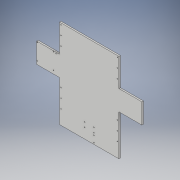
# Autodesk Inventor part: 20Gen2PlatePart
Saved by Autodesk Inventor 2019 (Build 230136000, 136)
## iProperties
Created: 2017-12-06
Part Number: 20Gen2PlatePart
Material: Generic
Document SubType Name: Modeling
Designer: User
Density: 1 g/cm^3
Appearance: Default
Mass: 688.034 g
Surface Area: 2294.14 cm^2
Volume: 688.034 cm^3
Author: User
Autodesk Inventor part; units mm, degrees
ref_plane "YZ Plane" through (0, 0, 0) normal (1, 0, 0) x (0, 1, 0)
ref_plane "XZ Plane" through (0, 0, 0) normal (0, 1, 0) x (-1, 0, 0)
ref_plane "XY Plane" through (0, 0, 0) normal (0, 0, 1) x (1, 0, 0)
ref_plane "Work Plane32" through (254, 330.2, 0) normal (0, 0, -1) x (-1, 0, 0)
sketch "Sketch36" plane through (254, 330.2, 0) normal (0, 0, -1) x (-1, 0, 0)
  line L0 (254, -363.855) -> (254, -196.85) projected
  line L1 (0, 0) -> (0, -114.3) projected
  line L2 (254, -363.855) -> (0, -363.855)
  line L3 (0, -363.855) -> (0, 0)
  line L4 (0, 0) -> (254, 0)
  line L5 (254, 0) -> (254, -363.855)
  line L6 (342.9, -196.85) -> (342.9, -114.3) projected
  line L7 (342.9, -196.85) -> (254, -196.85)
  line L8 (254, -196.85) -> (254, -114.3)
  line L9 (254, -114.3) -> (342.9, -114.3)
  line L10 (342.9, -114.3) -> (342.9, -196.85)
  line L11 (-31.75, -363.855) -> (254, -363.855) projected
  line L12 (0, -314.325) -> (0, -196.85) projected
  line L13 (-31.75, -363.855) -> (0, -363.855)
  line L14 (0, -363.855) -> (0, -314.325)
  line L15 (0, -314.325) -> (-31.75, -314.325)
  line L16 (-31.75, -314.325) -> (-31.75, -363.855)
  line L17 (0, -196.85) -> (-88.9, -196.85)
  line L18 (-88.9, -196.85) -> (-88.9, -114.3)
  line L19 (-88.9, -114.3) -> (0, -114.3)
  line L20 (0, -114.3) -> (0, -196.85)
  dimension "d412" = 82.55
  dimension "d413" = 254
  dimension "d414" = 31.75
  constraints: 32 end point, 8 parallel, 4 horizontal, 4 perpendicular, 1 point on line
  measures "d412" distance between parallel lines of L9 L7
  measures "d413" distance between parallel lines of L5 L1
  measures "d414" distance between parallel lines of L3 L16
extrude "Extrusion20" add sketch "Sketch36" along normal blind 6.35
ref_plane "Work Plane28" through (254, 330.2, -6.35) normal (0, 0, -1) x (-1, 0, 0)
sketch "Sketch38" plane through (254, 330.2, -6.35) normal (0, 0, -1) x (-1, 0, 0)
  circle A0 centre (273.685, -183.515) radius 1.778 projected
  circle A1 centre (273.685, -183.515) radius 1.778
  circle A2 centre (339.725, -183.515) radius 1.778 projected
  circle A3 centre (339.725, -183.515) radius 1.778
  circle A4 centre (339.725, -117.475) radius 1.778 projected
  circle A5 centre (339.725, -117.475) radius 1.778
  circle A6 centre (273.685, -117.475) radius 1.778 projected
  circle A7 centre (273.685, -117.475) radius 1.778
  circle A8 centre (263.1059, -119.0625) radius 1.778 projected
  circle A9 centre (263.1059, -119.0625) radius 1.778
  circle A10 centre (107.95, -332.105) radius 1.905 projected
  circle A11 centre (107.95, -332.105) radius 1.905
  circle A12 centre (107.95, -322.58) radius 1.905 projected
  circle A13 centre (107.95, -322.58) radius 1.905
  circle A14 centre (107.95, -303.53) radius 1.905 projected
  circle A15 centre (107.95, -303.53) radius 1.905
  circle A16 centre (107.95, -357.505) radius 1.905 projected
  circle A17 centre (107.95, -357.505) radius 1.905
  circle A18 centre (146.05, -303.53) radius 1.905 projected
  circle A19 centre (146.05, -303.53) radius 1.905
  circle A20 centre (146.05, -322.58) radius 1.905 projected
  circle A21 centre (146.05, -322.58) radius 1.905
  constraints: 11 centre point, 11 coincident
extrude "Extrusion21" cut sketch "Sketch38" against normal blind 6.35
sketch "Sketch39" plane through (254, 330.2, -6.35) normal (0, 0, -1) x (-1, 0, 0)
  line L0 (0, -196.85) -> (0, -314.325) projected
  line L1 (0, -196.85) -> (5.08, -196.85)
  line L2 (5.08, -196.85) -> (5.08, -314.325)
  line L3 (5.08, -314.325) -> (0, -314.325)
  line L4 (0, -314.325) -> (0, -196.85)
  line L5 (254, -363.855) -> (254, -196.85) projected
  line L6 (-31.75, -363.855) -> (254, -363.855) projected
  line L7 (254, -196.85) -> (248.92, -196.85)
  line L8 (248.92, -196.85) -> (248.92, -363.855)
  line L9 (248.92, -363.855) -> (254, -363.855)
  line L10 (254, -363.855) -> (254, -196.85)
  line L11 (0, -114.3) -> (-88.9, -114.3) projected
  line L12 (254, 0) -> (0, 0) projected
  line L13 (0, -114.3) -> (5.08, -114.3)
  line L14 (5.08, -114.3) -> (5.08, 0)
  line L15 (5.08, 0) -> (0, 0)
  line L16 (0, 0) -> (0, -114.3)
  line L17 (254, 0) -> (248.92, 0)
  line L18 (248.92, 0) -> (248.92, -114.3)
  line L19 (248.92, -114.3) -> (254, -114.3)
  line L20 (254, -114.3) -> (254, 0)
  point P0 (254, -330.2)
  dimension "d415" = 5.08
  dimension "d416" = 5.08
  dimension "d417" = 5.08
  constraints: 32 end point, 8 parallel, 4 horizontal, 4 perpendicular, 4 point on line
  measures "d415" distance of L2.end L3.end
  measures "d416" distance of L9.end L8.end
  measures "d417" distance of L15.end L14.end
extrude "Extrusion22" cut sketch "Sketch39" against normal blind 6.35
sketch "Sketch40" plane through (254, 330.2, -6.35) normal (0, 0, -1) x (-1, 0, 0)
  line L0 (5.08, 0) -> (5.08, -114.3) projected
  line L1 (248.92, 0) -> (5.08, 0) projected
  line L2 (248.92, -114.3) -> (248.92, 0) projected
  line L3 (-31.75, -363.855) -> (248.92, -363.855) projected
  line L4 (248.92, -363.855) -> (248.92, -196.85) projected
  circle A0 centre (11.43, -305.435) radius 1.778
  circle A1 centre (11.43, -267.335) radius 1.778
  circle A2 centre (11.43, -229.235) radius 1.778
  circle A3 centre (11.43, -82.55) radius 1.778
  circle A4 centre (11.43, -44.45) radius 1.778
  circle A5 centre (11.43, -6.35) radius 1.778
  circle A6 centre (242.57, -6.35) radius 1.778
  circle A7 centre (242.57, -44.45) radius 1.778
  circle A8 centre (242.57, -82.55) radius 1.778
  circle A9 centre (242.57, -229.235) radius 1.778
  circle A10 centre (242.57, -267.335) radius 1.778
  circle A11 centre (242.57, -305.435) radius 1.778
  point P0 (254, -330.2)
  dimension "d420" = 6.35
  dimension "d421" = 6.35
  dimension "d422" = 38.1
  dimension "d423" = 38.1
  dimension "d424" = 6.35
  dimension "d425" = 6.35
  dimension "d426" = 38.1
  dimension "d427" = 38.1
  dimension "d428" = 58.42
  dimension "d429" = 38.1
  dimension "d430" = 38.1
  dimension "d431" = 6.35
  dimension "d432" = 6.35
  dimension "d433" = 6.35
  dimension "d434" = 3.556
  dimension "d435" = 3.556
  dimension "d436" = 3.556
  dimension "d437" = 3.556
  dimension "d438" = 3.556
  dimension "d439" = 3.556
  dimension "d440" = 3.556
  dimension "d441" = 3.556
  dimension "d442" = 3.556
  dimension "d443" = 3.556
  dimension "d444" = 3.556
  dimension "d445" = 3.556
  constraints: 12 centre point, 12 coincident
  measures "d420" distance from line of L0 point (11.43, -6.35)
  measures "d421" distance from line of L1 point (11.43, -6.35)
  measures "d422" distance of point (11.43, -6.35) point (11.43, -44.45)
  measures "d423" distance of point (11.43, -44.45) point (11.43, -82.55)
  measures "d424" distance from line of L1 point (242.57, -6.35)
  measures "d425" distance from line of L2 point (242.57, -6.35)
  measures "d426" distance of point (242.57, -6.35) point (242.57, -44.45)
  measures "d427" distance of point (242.57, -44.45) point (242.57, -82.55)
  measures "d428" distance from line of L3 point (11.43, -305.435)
  measures "d429" distance of point (11.43, -267.335) point (11.43, -305.435)
  measures "d430" distance of point (11.43, -229.235) point (11.43, -267.335)
  measures "d431" distance from line of L4 point (242.57, -305.435)
  measures "d432" distance from line of L4 point (242.57, -267.335)
  measures "d433" distance from line of L4 point (242.57, -229.235)
  measures "d434" diameter of A0
  measures "d435" diameter of A1
  measures "d436" diameter of A2
  measures "d437" diameter of A3
  measures "d438" diameter of A4
  measures "d439" diameter of A5
  measures "d440" diameter of A6
  measures "d441" diameter of A7
  measures "d442" diameter of A8
  measures "d443" diameter of A9
  measures "d444" diameter of A10
  measures "d445" diameter of A11
extrude "Extrusion23" cut sketch "Sketch40" against normal blind 6.35
sketch "Sketch41" plane through (254, 330.2, 0) normal (0, 0, 1) x (1, 0, 0)
  line L0 (-5.08, -314.325) -> (31.75, -314.325) projected
  line L1 (31.75, -363.855) -> (-248.92, -363.855) projected
  line L2 (31.75, -314.325) -> (-5.08, -314.325)
  line L3 (-5.08, -314.325) -> (-5.08, -363.855)
  line L4 (-5.08, -363.855) -> (31.75, -363.855)
  line L5 (31.75, -363.855) -> (31.75, -314.325)
  point P0 (-254, -330.2)
  dimension "d448" = 36.83
  constraints: 8 end point, 2 parallel, 1 horizontal, 1 perpendicular, 1 point on line
  measures "d448" distance of L4.end L3.end
extrude "Extrusion24" cut sketch "Sketch41" against normal blind 6.35
body "Solid1"
